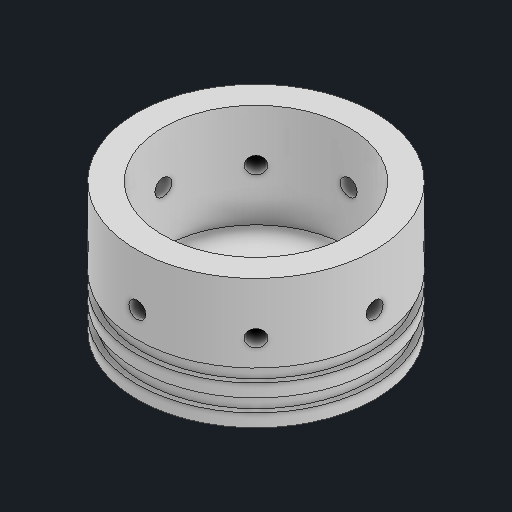
# Autodesk Inventor part: bulk head 94mm
Saved by Autodesk Inventor 2027 (Build 310192060, 192F)
## iProperties
Created: 2026-06-30
Part Number: bulk head 94mm
Material: Generic
Document SubType Name: Modeling
Designer: Alex T. Wandugu
Density: 1 g/cm^3
Appearance: Default
Matter: Aluminium
Author: Alex T. Wandugu
Autodesk Inventor part; units mm, degrees
ref_plane "YZ Plane" through (0, 0, 0) normal (1, 0, 0) x (0, 1, 0)
ref_plane "XZ Plane" through (0, 0, 0) normal (0, 1, 0) x (-1, 0, 0)
sketch "Sketch1" plane through (0, 0, 0) normal (0, 1, 0) x (-1, 0, 0)
  circle A0 centre (0, 0) radius 46
  dimension "d0" = 92
  constraints: 1 centre point, 1 coincident
  measures "d0" diameter of A0
extrude "Extrusion1" add sketch "Sketch1" along normal blind 50
ref_plane "Work Plane1" through (0, 50, 0) normal (0, 1, 0) x (1, 0, 0)
sketch "Sketch2" plane through (0, 50, 0) normal (0, 1, 0) x (1, 0, 0)
  circle A0 centre (0, 0) radius 36
  dimension "d4" = 72
  constraints: 1 centre point, 1 coincident
  measures "d4" diameter of A0
extrude "Extrusion2" cut sketch "Sketch2" against normal blind 40
sketch "Sketch3" plane through (0, 0, 0) normal (1, 0, 0) x (0, 1, 0)
  line L0 (50, -46) -> (0, -46) projected
  line L1 (0, -46) -> (0, 46) projected
  line L2 (0, 46) -> (50, 46) projected
  line L3 (50, 46) -> (50, 36) projected
  line L4 (50, 36) -> (10, 36) projected
  line L5 (10, 36) -> (10, -36) projected
  line L6 (10, -36) -> (50, -36) projected
  line L7 (50, -36) -> (50, -46) projected
  line L8 (0, 46) -> (50, 46) projected
  line L9 (10, 46) -> (5, 46)
  line L10 (5, 46) -> (5, 44)
  line L11 (5, 44) -> (10, 44)
  line L12 (10, 44) -> (10, 46)
  line L13 (20, 46) -> (15, 46)
  line L14 (15, 46) -> (15, 44)
  line L15 (15, 44) -> (20, 44)
  line L16 (20, 44) -> (20, 46)
  line L17 (-10, 0) -> (60, 0) projected
  point P0 (0, 0)
  point P1 (15, 46)
  dimension "d7" = 5
  dimension "d8" = 5
  dimension "d9" = 5
  dimension "d10" = 5
  dimension "d11" = 2
  constraints: 16 end point, 7 point on line, 4 parallel, 2 horizontal, 2 perpendicular
  measures "d7" distance of L8.start point (5, 46)
  measures "d8" distance of L9.start point (5, 46)
  measures "d9" distance of L9.start point (15, 46)
  measures "d10" distance of point (15, 46) L13.start
  measures "d11" distance of L10.end L9.end
revolve "Revolution1" cut sketch "Sketch3" angle 360 about axis through (0, -10, 0) along (0, 1, 0) contours L2 L12 L11 L10 | L2 L16 L15 L14
sketch "Sketch4" plane through (0, 0, 0) normal (1, 0, 0) x (0, 1, 0)
  line L0 (10, -36) -> (50, -36) projected
  line L1 (50, -36) -> (50, -46) projected
  line L2 (50, -46) -> (20, -46) projected
  line L3 (20, -46) -> (20, -44) projected
  line L4 (20, -44) -> (15, -44) projected
  line L5 (15, -44) -> (15, -46) projected
  line L6 (15, -46) -> (10, -46) projected
  line L7 (10, -46) -> (10, -44) projected
  line L8 (10, -44) -> (5, -44) projected
  line L9 (5, -44) -> (5, -46) projected
  line L10 (5, -46) -> (0, -46) projected
  line L11 (0, -46) -> (0, 46) projected
  line L12 (0, 46) -> (5, 46) projected
  line L13 (5, 46) -> (5, 44) projected
  line L14 (5, 44) -> (10, 44) projected
  line L15 (10, 44) -> (10, 46) projected
  line L16 (10, 46) -> (15, 46) projected
  line L17 (15, 46) -> (15, 44) projected
  line L18 (15, 44) -> (20, 44) projected
  line L19 (20, 44) -> (20, 46) projected
  line L20 (20, 46) -> (50, 46) projected
  line L21 (50, 46) -> (50, 36) projected
  line L22 (50, 36) -> (10, 36) projected
  line L23 (10, 36) -> (10, -36) projected
  line L24 (10, -36) -> (50, -36) projected
  line L25 (50, -36) -> (50, -46) projected
  line L26 (50, 46) -> (50, 36) projected
  line L27 (50, 36) -> (10, 36) projected
  line L28 (10, 36) -> (10, -36) projected
  line L29 (20, -46) -> (20, 46) projected
  line L30 (50, -46) -> (50, 46) projected
  circle A0 centre (30, 0) radius 3.25
  line L31 (50, -46) -> (20, -46) projected
  line L32 (20, -46) -> (20, -44) projected
  line L33 (20, -44) -> (15, -44) projected
  line L34 (15, -44) -> (15, -46) projected
  line L35 (15, -46) -> (10, -46) projected
  line L36 (10, -46) -> (10, -44) projected
  line L37 (10, -44) -> (5, -44) projected
  line L38 (5, -44) -> (5, -46) projected
  line L39 (5, -46) -> (0, -46) projected
  line L40 (0, -46) -> (0, 46) projected
  line L41 (0, 46) -> (5, 46) projected
  line L42 (5, 46) -> (5, 44) projected
  line L43 (5, 44) -> (10, 44) projected
  line L44 (10, 44) -> (10, 46) projected
  line L45 (10, 46) -> (15, 46) projected
  line L46 (15, 46) -> (15, 44) projected
  line L47 (15, 44) -> (20, 44) projected
  line L48 (20, 44) -> (20, 46) projected
  line L49 (20, 46) -> (50, 46) projected
  point P0 (0, 0)
  dimension "d17" = 6.5
  dimension "d18" = 20
  constraints: 1 centre point
  measures "d17" diameter of A0
  measures "d18" distance from line of A0.centre L30
extrude "Extrusion3" cut sketch "Sketch4" along normal through all both and the other way through all contours A0
pattern_circular "Circular Pattern1" count 8 over 360 about axis through (0, 50, 0) along (0, -1, 0) of "Extrusion3"
body "Solid1"
